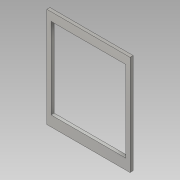
# Autodesk Inventor part: Left Face
Saved by Autodesk Inventor 2016 (Build 200138000, 138)
## iProperties
Created: 2017-05-17
Part Number: Left Face
Material: Generic
Document SubType Name: Modeling
Designer: 31745
Density: 1 g/cm^3
Appearance: Default
Author: 31745
Autodesk Inventor part; units mm, degrees
ref_plane "YZ Plane" through (0, 0, 0) normal (1, 0, 0) x (0, 1, 0)
ref_plane "XZ Plane" through (0, 0, 0) normal (0, 1, 0) x (-1, 0, 0)
ref_plane "XY Plane" through (0, 0, 0) normal (0, 0, 1) x (1, 0, 0)
sketch "Sketch1" plane through (0, 0, 0) normal (0, 0, 1) x (1, 0, 0)
  line L0 (0, 0) -> (254, 0)
  line L1 (254, 0) -> (254, 304.8)
  line L2 (254, 304.8) -> (0, 304.8)
  line L3 (0, 304.8) -> (0, 0)
  dimension "d0" = 254
  dimension "d1" = 304.8
  constraints: 8 end point, 2 parallel, 1 horizontal, 1 perpendicular
  measures "d0" distance of L2.end L1.end
  measures "d1" distance of L1.end L0.end
extrude "Extrusion1" add sketch "Sketch1" against normal blind 9.525
sketch "Sketch2" plane through (0, 0, 0) normal (0, 0, 1) x (1, 0, 0)
  line L0 (12.7, 279.4) -> (241.3, 279.4)
  line L1 (241.3, 279.4) -> (241.3, 31.75)
  line L2 (241.3, 31.75) -> (12.7, 31.75)
  line L3 (12.7, 31.75) -> (12.7, 279.4)
  line L4 (0, 0) -> (254, 0) projected
  line L5 (254, 0) -> (254, 304.8) projected
  line L6 (254, 304.8) -> (0, 304.8) projected
  line L7 (0, 304.8) -> (0, 0) projected
  point P0 (127, 279.4)
  point P1 (127, 304.8)
  dimension "d4" = 25.4
  dimension "d5" = 31.75
  dimension "d6" = 12.7
  constraints: 8 end point, 2 midpoint, 2 parallel, 1 horizontal, 1 perpendicular, 1 vertical alignment
  measures "d4" distance between parallel lines of L6 L0
  measures "d5" distance between parallel lines of L4 L2
  measures "d6" distance between parallel lines of L5 L1
extrude "Extrusion2" cut sketch "Sketch2" against normal through all contours L0 L1 L2 L3
body "Solid1"
